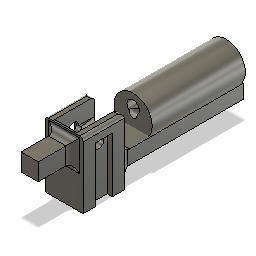
Nectary Stand with front slit- straight hole for flower open IR v2 (Autodesk Fusion 360 design; units mm, degrees)
Autodesk Fusion 360 part; units mm, degrees
note: some values were not read from the file. Chosen so that the rebuilt part matches the saved one: which face or edge a step refers to; which pieces of a blend or face edit are solid. Set by a fixed rule: which sketch regions a step uses.
sketch "Base Rod" plane through (0, 0, 0) normal (0, 1, 0) x (1, 0, 0)
  line L0 (0, 17.5) -> (10, 17.5)
  line L1 (10, 17.5) -> (10, -17.5)
  line L2 (10, -17.5) -> (0, -17.5)
  line L3 (0, -17.5) -> (0, 17.5)
  dimension "d1" = 10
  dimension "d2" = 35
extrude "Extrude1" add sketch "Base Rod" along normal blind 4 makes body 1
sketch "adapter for holding flowe facade" plane through (0, 0, -17.5) normal (0, 0, -1) x (-1, 0, 0)
  line L0 (-10, 0) -> (0, 0)
  line L1 (0, 0) -> (0, 4)
  line L2 (0, 4) -> (-10, 4)
  line L3 (-10, 4) -> (-10, 0)
  line L4 (-5, 0) -> (-5, 4) construction
  line L5 (-10, 2) -> (0, 2) construction
  line L6 (-5, 4) -> (-5, 7) construction
  circle A0 centre (-5, 7) radius 5.5
  dimension "d6" = 3
  dimension "d7" = 11
  measures "d7" diameter of A0
extrude "Extrude2" add sketch "adapter for holding flowe facade" against normal blind 27 separate body contours L2 A0 | L2 A0 makes body 2
sketch "top hole for facade" plane through (0, 0, -17.5) normal (0, 0, -1) x (-1, 0, 0)
  circle A0 centre (-5, 7) radius 5.5
  circle A1 centre (-5, 9) radius 2.75
  line L0 (0, 4) -> (-10, 4)
  line L1 (-5, 4) -> (-5, 9) construction
  dimension "d12" = 5.5
  dimension "d222" = 5
  measures "d12" diameter of A1
ref_plane "WorkPlane10" through (5, 9.1448, -13.5) normal (0, 0, -1) x (-1, 0, 0)
sketch "top hole for flower taper" plane through (5, 9.1448, -13.5) normal (0, 0, -1) x (1, 0, 0)
  circle A0 centre (0, 0.1448) radius 2.75
  dimension "d221" = 5.5
  measures "d221" diameter of A0
extrude "Extrude21" [suppressed]
sketch "taper for flower facade" plane through (0, 0, 9.5) normal (0, 0, 1) x (1, 0, 0)
  circle A0 centre (5, 7) radius 5.5
  circle A1 centre (5, 9) radius 1.8
  dimension "d95" = 3.6
  measures "d95" diameter of A1
loft "Loft7" cut profiles "taper for flower facade", "top hole for facade" section 1 contours A1 section 2 contours A1 bodies 2
sketch "IR and nectary tube base" plane through (0, 0, 0) normal (0, 1, 0) x (1, 0, 0)
  line L0 (12, -17.5) -> (-2, -17.5)
  line L1 (-2, -17.5) -> (-2, -29.5)
  line L2 (-2, -29.5) -> (12, -29.5)
  line L3 (12, -29.5) -> (12, -17.5)
  line L4 (10, -17.5) -> (0, -17.5)
  dimension "d20" = 14
  dimension "d21" = 12
extrude "Extrude4" add sketch "IR and nectary tube base" along normal blind 14 and the other way blind 5 bodies 1
sketch "top for nectar tube holder" plane through (5, 9, 17.5) normal (0, 0, -1) x (1, 0, 0)
  circle A0 centre (0, 0) radius 3.25
  line L0 (-7, 14) -> (-7, -5)
  line L1 (-7, -5) -> (7, -5)
  line L2 (7, -5) -> (7, 14)
  line L3 (7, 14) -> (-7, 14)
  line L4 (5, 9) -> (5, 5)
  line L5 (5, 5) -> (-5, 5)
  line L6 (-5, 5) -> (-5, 9)
  line L7 (-5, 9) -> (5, 9)
  dimension "d27" = 6.5
  measures "d27" diameter of A0
sketch "bottom for nectar tube holder" plane through (5, 9, 29.5) normal (0, 0, 1) x (1, 0, 0)
  circle A0 centre (0, 0) radius 1.5
  line L0 (7, -14) -> (7, 5)
  line L1 (7, 5) -> (-7, 5)
  line L2 (-7, 5) -> (-7, -14)
  line L3 (-7, -14) -> (7, -14)
  dimension "d30" = 3
  measures "d30" diameter of A0
loft "Loft2" cut profiles "top for nectar tube holder", "bottom for nectar tube holder" section 1 contours A0 section 2 contours A0 bodies 1
sketch "front slit" plane through (0, 14, 0) normal (0, 1, 0) x (-1, 0, 0)
  line L0 (-12, 17.5) -> (2, 17.5)
  line L1 (2, 17.5) -> (2, 29.5)
  line L2 (2, 29.5) -> (-12, 29.5)
  line L3 (-12, 29.5) -> (-12, 17.5)
  line L4 (-5, 29.5) -> (-5, 29) construction
  line L5 (-1.75, 29) -> (-8.25, 29) construction
  line L6 (-1.75, 29) -> (-8.25, 29)
  line L7 (-8.25, 29) -> (-8.25, 17.5)
  line L8 (-8.25, 17.5) -> (-1.75, 17.5)
  line L9 (-1.75, 17.5) -> (-1.75, 29)
  dimension "d213" = 0.5
  dimension "d214" = 6.5
extrude "Extrude20" cut sketch "front slit" against normal blind 5 contours L0 L6 L7 L8 L9 bodies 1
sketch "bottom rod to coonect to 80-20 connector" plane through (5, 9, 29.5) normal (0, 0, 1) x (1, 0, 0)
  line L0 (2.5, 2.5) -> (-2.5, 2.5)
  line L1 (-2.5, 2.5) -> (-2.5, -2.5)
  line L2 (-2.5, -2.5) -> (2.5, -2.5)
  line L3 (2.5, -2.5) -> (2.5, 2.5)
  line L4 (2.5, 2.5) -> (-2.5, -2.5) construction
  line L5 (-2.5, 2.5) -> (2.5, -2.5) construction
  circle A0 centre (0, 0) radius 1.5
  line L6 (7, -14) -> (7, 5)
  line L7 (7, 5) -> (-7, 5)
  line L8 (-7, 5) -> (-7, -14)
  line L9 (-7, -14) -> (7, -14)
  dimension "d56" = 5
  dimension "d57" = 5
extrude "Extrude9" add sketch "bottom rod to coonect to 80-20 connector" along normal blind 10 contours L0 L1 L2 L3 | A0 bodies 1
extrude "Extrude10" cut 1 faces at (5.2179, 9.3289, 29.5) along direction (0, 0, 1) blind 2 on bodies 1 bodies 1
sketch "IR sensor holder" plane through (12, 0, 0) normal (1, 0, 0) x (0, 0, -1)
  line L0 (-23.5, 14) -> (-23.5, 9) construction
  circle A0 centre (-23.5, 9) radius 1.5
  line L1 (-23.5, 9) -> (-23.5, 10.5)
  line L2 (-21.75, 7.5) -> (-25.25, 7.5)
  line L3 (-25.25, 7.5) -> (-25.25, 10.5)
  line L4 (-25.25, 10.5) -> (-21.75, 10.5)
  line L5 (-21.75, 10.5) -> (-21.75, 7.5)
  line L6 (-21.75, 7.5) -> (-25.25, 10.5) construction
  line L7 (-25.25, 7.5) -> (-21.75, 10.5) construction
  line L8 (-23.5, 9) -> (-23.5, 11)
  line L9 (-26, 11) -> (-21, 11)
  line L10 (-21, 11) -> (-21, -5)
  line L11 (-21, -5) -> (-26, -5)
  line L12 (-26, -5) -> (-26, 11)
  line L13 (-17.5, -5) -> (-17.5, 14)
  line L14 (-17.5, 14) -> (-29.5, 14)
  line L15 (-29.5, 14) -> (-29.5, -5)
  line L16 (-29.5, -5) -> (-17.5, -5)
  line L17 (-17.5, -5) -> (-17.5, 14)
  line L18 (-17.5, 14) -> (-29.5, 14)
  line L19 (-29.5, 14) -> (-29.5, -5)
  line L20 (-29.5, -5) -> (-17.5, -5)
  line L21 (-17.5, -5) -> (-17.5, 14)
  line L22 (-17.5, 14) -> (-29.5, 14)
  line L23 (-29.5, 14) -> (-29.5, -5)
  line L24 (-29.5, -5) -> (-17.5, -5)
  dimension "d40" = 3
  dimension "d97" = 5
  dimension "d111" = 1.5
  dimension "d112" = 3.5
  dimension "d113" = 2
  dimension "d115" = 5
  measures "d40" diameter of A0
extrude "Extrude11" cut sketch "IR sensor holder" against normal up to surface (14 mm away) contours A0 bodies 1
extrude "Extrude13" cut sketch "IR sensor holder" against normal blind 3 contours A0 L2 L4 L5 | A0 L2 L3 L4 | L9 L10 L11 L12 L16 L20 L24 bodies 1
extrude "Extrude22" cut 1 faces at (12, 6.6667, 18.6667) along direction (-1, 0, 0) blind 1.5 on bodies 1 bodies 1
ref_plane "WorkPlane6" through (5, 4.5, 23.5) normal (1, 0, 0) x (0, 0, -1)
mirror "Mirror3" about plane through (5, 4.5, 23.5) normal (1, 0, 0) of "Extrude13", "Extrude22"
sketch "pipe for nectary" plane through (5, 7.5, 27.5) normal (1, 0, 0) x (0, 0, -1)
  line L0 (10, -3.5) -> (10, 1.5) construction
  line L1 (10, 1.5) -> (17, 1.5) construction
  line L2 (17, 1.5) -> (33.9706, -15.4706)
  line L3 (17, 1.5) -> (33, 1.5) construction
  line L4 (17, 1.5) -> (26.8284, 1.5) construction
  line L5 (24.25, -5.75) -> (17, 1.5)
  dimension "d100" = 5
  dimension "d101" = 45
  dimension "d102" = 24
  dimension "d108" = 7
  measures "d101" angle of L2 L3
pipe "Pipe10" cut diameter 2.5 path "pipe for nectary" along L2 bodies 1 2
fillet "Fillet3" radius 2 4 edges at (10, 2, 17.5) (5, 0, 17.5) (5, 4, 17.5) (0, 2, 17.5) on bodies 1
fillet "Fillet4" radius 2 4 edges at (5, 6.5, 29.5) (2.5, 9, 29.5) (5, 11.5, 29.5) (7.5, 9, 29.5) on bodies 1
fillet "Fillet7" radius 1 4 edges at (0.625, 14, 17.5) (9.375, 14, 17.5) (10.5, 14, 23.5) (-0.5, 14, 23.5) on bodies 1
